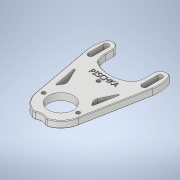
# Autodesk Inventor part: Motor Holder v3
Saved by Autodesk Inventor 2020.1 (Build 241239000, 239)
## iProperties
Created: 2019-03-01
Part Number: Motor Holder v3
Material: ABS Plastic
Document SubType Name: Modeling
Designer: Petar
Density: 1.06 g/cm^3
Appearance: Smooth - White
Mass: 12.2882 g
Surface Area: 69.5635 cm^2
Volume: 11.5927 cm^3
Author: Petar
Autodesk Inventor part; units mm, degrees
ref_plane "YZ Plane" through (0, 0, 0) normal (1, 0, 0) x (0, 1, 0)
ref_plane "XZ Plane" through (0, 0, 0) normal (0, 1, 0) x (-1, 0, 0)
ref_plane "XY Plane" through (0, 0, 0) normal (0, 0, 1) x (1, 0, 0)
sketch "Sketch1" plane through (0, 0, 0) normal (0, 1, 0) x (-1, 0, 0)
  line L0 (0, 0) -> (0, 51.5) construction
  circle A0 centre (0, 51.5) radius 10
  line L1 (16, -6.25) -> (16, 0)
  line L2 (21.5, 19.889372) -> (21.5, -14.110628) construction
  line L3 (-21.5, 18) -> (-21.5, -16) construction
  circle A1 centre (21.5, 3.5) radius 1.75 construction
  circle A2 centre (21.5, -3.5) radius 1.75 construction
  circle A3 centre (-21.5, 3.5) radius 1.75 construction
  circle A4 centre (-21.5, -3.5) radius 1.75 construction
  line L4 (-16, -6.25) -> (-16, 0)
  line L5 (21.5, 6.25) -> (21.5, -6.25) construction
  line L6 (19.45, 6.25) -> (19.45, -6.25)
  line L7 (23.55, -6.25) -> (23.55, 6.25)
  arc A5 (23.55, 6.25) -> (19.45, 6.25) centre (21.5, 6.25) ccw
  arc A6 (19.45, -6.25) -> (23.55, -6.25) centre (21.5, -6.25) ccw
  line L8 (-19.45, 6.25) -> (-19.45, -6.25)
  line L9 (-23.55, -6.25) -> (-23.55, 6.25)
  arc A7 (-19.45, 6.25) -> (-23.55, 6.25) centre (-21.5, 6.25) ccw
  arc A8 (-23.55, -6.25) -> (-19.45, -6.25) centre (-21.5, -6.25) ccw
  arc A9 (14.544724, 41.768556) -> (17.199681, 54.728155) centre (0, 51.5) ccw construction
  arc A10 (16, -6.25) -> (24.816002, -10.637953) centre (21.5, -6.25) ccw
  arc A11 (-24.816002, -10.637953) -> (-16, -6.25) centre (-21.5, -6.25) ccw
  line L10 (17.199681, 54.728155) -> (26.53665, 4.980583)
  line L11 (-17.199681, 54.728155) -> (-26.53665, 4.980583)
  circle A12 centre (0, 51.5) radius 13.75 construction
  circle A13 centre (9.722718, 61.222718) radius 1.5 construction
  circle A14 centre (9.722718, 41.777282) radius 1.5 construction
  line L12 (0, 51.5) -> (9.722718, 61.222718) construction
  line L13 (9.722718, 41.777282) -> (0, 51.5) construction
  circle A15 centre (-9.722718, 61.222718) radius 1.5 construction
  circle A16 centre (-9.722718, 41.777282) radius 1.5 construction
  circle A17 centre (13.75, 51.5) radius 1.5
  line L14 (13.75, 51.5) -> (0, 51.5) construction
  circle A18 centre (-13.75, 51.5) radius 1.5
  circle A19 centre (0, 21.442114) radius 1.5
  line L15 (14.544724, 41.768556) -> (18.735106, 19.442114)
  arc A20 (17.199681, 54.728155) -> (-17.199681, 54.728155) centre (0, 51.5) ccw
  arc A21 (-17.199681, 54.728155) -> (-14.544724, 41.768556) centre (0, 51.5) ccw construction
  line L16 (-14.544724, 41.768556) -> (-18.735106, 19.442114)
  line L17 (5, 68.27051) -> (0, 65.25) construction
  line L18 (0, 65.25) -> (-5, 68.27051) construction
  spline S0 degree 2 poles (5, 68.27051) (0, 65.25) (-5, 68.27051) knots 1 1 1 2 2 2
  line L19 (5, 68.27051) -> (-5, 68.27051) construction
  line L20 (18.735106, 19.442114) -> (-18.735106, 19.442114) construction
  line L21 (18.735106, 19.442114) -> (11.806239, 33.884362)
  line L22 (14.544724, 41.768556) -> (12.108743, 38.127711)
  arc A22 (12.108743, 38.127711) -> (11.806239, 33.884362) centre (15.676028, 35.740946) ccw
  line L23 (-18.735106, 19.442114) -> (-11.806239, 33.884362)
  line L24 (-14.544724, 41.768556) -> (-12.108743, 38.127711)
  arc A23 (-11.806239, 33.884362) -> (-12.108743, 38.127711) centre (-15.676028, 35.740946) ccw
  line L25 (14.298579, 19.442114) -> (8.163141, 32.230571) construction
  line L26 (14.298579, 19.442114) -> (7.49461, 25.938983) construction
  line L27 (8.163141, 32.230571) -> (6.995239, 30.485011) construction
  arc A24 (6.995239, 30.485011) -> (7.49461, 25.938983) centre (9.94862, 28.508992) ccw construction
  line L28 (-14.298579, 19.442114) -> (-8.163141, 32.230571) construction
  line L29 (-14.298579, 19.442114) -> (-7.49461, 25.938983) construction
  line L30 (-8.163141, 32.230571) -> (-6.995239, 30.485011) construction
  arc A25 (-7.49461, 25.938983) -> (-6.995239, 30.485011) centre (-9.94862, 28.508992) ccw construction
  arc A26 (24.816002, -10.637953) -> (27, 0) centre (0, 0) ccw
  arc A27 (-24.816002, -10.637953) -> (24.816002, -10.637953) centre (0, 0) ccw construction
  arc A28 (-10.270866, 24.970168) -> (-26.53665, 4.980583) centre (0, 0) ccw construction
  line L31 (21.5, -11.75) -> (-21.5, -11.75) construction
  line L32 (-21.213203, 69) -> (25, 69) construction
  line L33 (0, 65.25) -> (0, 61.5) construction
  arc A29 (13.760985, 8.163043) -> (-13.760985, 8.163043) centre (0, -11.5) ccw
  line L34 (13.760985, 8.163043) -> (-13.760985, 8.163043) construction
  arc A30 (16, 0) -> (13.760985, 8.163043) centre (0, 0) ccw
  arc A31 (-13.760985, 8.163043) -> (-16, 0) centre (0, 0) ccw
  arc A32 (27, 0) -> (26.53665, 4.980583) centre (0, 0) ccw
  arc A33 (-27, 0) -> (-24.816002, -10.637953) centre (0, 0) ccw
  arc A34 (-26.53665, 4.980583) -> (-27, 0) centre (0, 0) ccw
  arc A35 (26.53665, 4.980583) -> (-12.029232, 24.172248) centre (0, 0) ccw construction
  line L35 (16, 0) -> (-16, 0) construction
  point P0 (21.5, 0)
  point P1 (0, 12.5)
  dimension "d1" = 20
  dimension "d0" = 51.5
  dimension "d3" = 3.5
  dimension "d4" = 3.5
  dimension "d5" = 7
  dimension "d9" = 3.5
  dimension "d11" = 32
  dimension "d15" = 4.1
  dimension "d24" = 3
  dimension "d25" = 3
  dimension "d27" = 45
  dimension "d29" = 3
  dimension "d30" = 3
  dimension "d50" = 10
  dimension "d53" = 27
  dimension "d75" = 80.75
  dimension "d76" = 7.5
  dimension "d77" = 3.75
  dimension "d81" = 6.25
  dimension "d82" = 12.5
  dimension "d85" = 5
  dimension "d86" = 4
  dimension "d98" = 15
  dimension "d99" = 24
  dimension "d102" = 43
  dimension "d103" = 2
  constraints: 70 end point, 59 point on circle, 35 centre point, 26 symmetric about line, 19 tangent, 13 point on line, 7 coincident, 5 horizontal, 5 vertical, 3 parallel, 2 perpendicular, 1 collinear, 1 midpoint, 1 vertical alignment, 16 other
  measures "d0" distance of L0.start L0.end
  measures "d3" diameter of A1
  measures "d4" diameter of A2
  measures "d5" distance of A2.centre A1.centre
  measures "d9" vertical distance of L0.start A1.centre
  measures "d11" distance between parallel lines of L4 L1
  measures "d15" distance between parallel lines of L6 L7
  measures "d24" diameter of A13
  measures "d25" diameter of A14
  measures "d27" angle of L0 L13
  measures "d29" diameter of A17
  measures "d30" diameter of A19
  measures "d50" distance of L17.start L18.end
  measures "d53" radius of A26
  measures "d75" distance between parallel lines of L31 L32
  measures "d81" vertical distance of L5.start point (0, 12.5)
  measures "d82" distance of L5.end L5.start
  measures "d85" distance between parallel lines of L10 L15
  measures "d86" distance between parallel lines of L21 L25
  measures "d98" angle of L15 L21
  measures "d99" radius of A29
  measures "d102" distance of A4.centre A2.centre
  measures "d103" distance from line of A19.centre L20
extrude "Extrusion3" add sketch "Sketch1" along normal blind 5.5 contours L1 A30 A29 A31 L4 A11 A33 A34 L11 A20 S0 L10 A32 A26 A10
thread "Thread1" size "M3x0.5" class "6H" standard "ANSI Metric M Profile" full length
thread "Thread2" size "M3x0.5" class "6H" standard "ANSI Metric M Profile" full length
thread "Thread3" size "M3x0.5" class "6H" standard "ANSI Metric M Profile" full length
sketch "Sketch3" plane through (0, 5.5, 0) normal (0, 1, 0) x (1, 0, 0)
  line L0 (-12.5, -14.442114) -> (12.5, -14.442114) construction
  line L1 (12.5, -14.442114) -> (12.5, -19.442114) construction
  line L2 (12.5, -19.442114) -> (-12.5, -19.442114) construction
  line L3 (-12.5, -19.442114) -> (-12.5, -14.442114) construction
  line L4 (0, 0) -> (0, -51.5) construction
  circle A0 centre (0, -21.442114) radius 1.5
  circle A1 centre (0, -51.5) radius 10 construction
  arc A2 (-24.816002, 10.637953) -> (-26.53665, -4.980583) centre (0, 0) ccw construction
  spline S0 degree 2 poles (-7.943274, -16.147949) (-7.943274, -16.407268) (-8.128039, -16.874043) (-8.293355, -17.036118) knots 0 0 0 1 2 2 2
  spline S1 degree 2 poles (-8.293355, -17.036118) (-8.500811, -17.240332) (-9.061589, -17.451029) (-9.489465, -17.451029) knots 0 0 0 1 2 2 2
  line L5 (-9.489465, -17.451029) -> (-9.940033, -17.451029)
  line L6 (-9.940033, -17.451029) -> (-9.940033, -18.942114)
  line L7 (-9.940033, -18.942114) -> (-10.471637, -18.942114)
  line L8 (-10.471637, -18.942114) -> (-10.471637, -14.942114)
  line L9 (-10.471637, -14.942114) -> (-9.466775, -14.942114)
  spline S2 degree 2 poles (-9.466775, -14.942114) (-9.110211, -14.942114) (-8.611021, -15.058808) (-8.419773, -15.191709) knots 0 0 0 1 2 2 2
  spline S3 degree 2 poles (-8.419773, -15.191709) (-8.19611, -15.344059) (-7.943274, -15.814076) (-7.943274, -16.147949) knots 0 0 0 1 2 2 2
  spline S4 degree 2 poles (-8.497569, -16.164157) (-8.497569, -15.956701) (-8.640195, -15.652001) (-8.786062, -15.554756) knots 0 0 0 1 2 2 2
  spline S5 degree 2 poles (-8.786062, -15.554756) (-8.91248, -15.470477) (-9.249595, -15.402406) (-9.49919, -15.402406) knots 0 0 0 1 2 2 2
  line L10 (-9.49919, -15.402406) -> (-9.940033, -15.402406)
  line L11 (-9.940033, -15.402406) -> (-9.940033, -16.99722)
  line L12 (-9.940033, -16.99722) -> (-9.576986, -16.99722)
  spline S6 degree 2 poles (-9.576986, -16.99722) (-9.252837, -16.99722) (-8.854133, -16.893492) (-8.724474, -16.757349) knots 0 0 0 1 2 2 2
  spline S7 degree 2 poles (-8.724474, -16.757349) (-8.604538, -16.637414) (-8.497569, -16.355405) (-8.497569, -16.164157) knots 0 0 0 1 2 2 2
  line L13 (-6.04376, -18.942114) -> (-7.593193, -18.942114)
  line L14 (-7.593193, -18.942114) -> (-7.593193, -18.533687)
  line L15 (-7.593193, -18.533687) -> (-7.084279, -18.533687)
  line L16 (-7.084279, -18.533687) -> (-7.084279, -15.350542)
  line L17 (-7.084279, -15.350542) -> (-7.593193, -15.350542)
  line L18 (-7.593193, -15.350542) -> (-7.593193, -14.942114)
  line L19 (-7.593193, -14.942114) -> (-6.04376, -14.942114)
  line L20 (-6.04376, -14.942114) -> (-6.04376, -15.350542)
  line L21 (-6.04376, -15.350542) -> (-6.552674, -15.350542)
  line L22 (-6.552674, -15.350542) -> (-6.552674, -18.533687)
  line L23 (-6.552674, -18.533687) -> (-6.04376, -18.533687)
  line L24 (-6.04376, -18.533687) -> (-6.04376, -18.942114)
  spline S8 degree 2 poles (-4.270665, -19.013427) (-4.705025, -19.013427) (-5.314425, -18.831904) (-5.583469, -18.702244) knots 0 0 0 1 2 2 2
  line L25 (-5.583469, -18.702244) -> (-5.583469, -18.034497)
  line L26 (-5.583469, -18.034497) -> (-5.544571, -18.034497)
  spline S9 degree 2 poles (-5.544571, -18.034497) (-5.28201, -18.28085) (-4.617504, -18.553136) (-4.309563, -18.553136) knots 0 0 0 1 2 2 2
  spline S10 degree 2 poles (-4.309563, -18.553136) (-3.86872, -18.553136) (-3.418153, -18.186847) (-3.418153, -17.885388) knots 0 0 0 1 2 2 2
  spline S11 degree 2 poles (-3.418153, -17.885388) (-3.418153, -17.645518) (-3.654781, -17.347301) (-3.910859, -17.272747) knots 0 0 0 1 2 2 2
  spline S12 degree 2 poles (-3.910859, -17.272747) (-4.095624, -17.220883) (-4.403566, -17.14957) (-4.633712, -17.091223) knots 0 0 0 1 2 2 2
  spline S13 degree 2 poles (-4.633712, -17.091223) (-4.841167, -17.036118) (-5.168558, -16.870802) (-5.294976, -16.7379) knots 0 0 0 1 2 2 2
  spline S14 degree 2 poles (-5.294976, -16.7379) (-5.418153, -16.604999) (-5.554295, -16.248435) (-5.554295, -16.015048) knots 0 0 0 1 2 2 2
  spline S15 degree 2 poles (-5.554295, -16.015048) (-5.554295, -15.528824) (-4.795786, -14.870802) (-4.209076, -14.870802) knots 0 0 0 1 2 2 2
  spline S16 degree 2 poles (-4.209076, -14.870802) (-3.871961, -14.870802) (-3.275527, -15.003703) (-3.019449, -15.130121) knots 0 0 0 1 2 2 2
  line L27 (-3.019449, -15.130121) -> (-3.019449, -15.765453)
  line L28 (-3.019449, -15.765453) -> (-3.058347, -15.765453)
  spline S17 degree 2 poles (-3.058347, -15.765453) (-3.249595, -15.590413) (-3.846029, -15.331093) (-4.17342, -15.331093) knots 0 0 0 1 2 2 2
  spline S18 degree 2 poles (-4.17342, -15.331093) (-4.54295, -15.331093) (-5, -15.677933) (-5, -15.959943) knots 0 0 0 1 2 2 2
  spline S19 degree 2 poles (-5, -15.959943) (-5, -16.212779) (-4.730956, -16.514238) (-4.47812, -16.582309) knots 0 0 0 1 2 2 2
  spline S20 degree 2 poles (-4.47812, -16.582309) (-4.309563, -16.62769) (-3.820097, -16.744383) (-3.658023, -16.793006) knots 0 0 0 1 2 2 2
  spline S21 degree 2 poles (-3.658023, -16.793006) (-3.246354, -16.919424) (-2.863858, -17.428338) (-2.863858, -17.80111) knots 0 0 0 1 2 2 2
  spline S22 degree 2 poles (-2.863858, -17.80111) (-2.863858, -18.037738) (-3.055106, -18.491547) (-3.226905, -18.65038) knots 0 0 0 1 2 2 2
  spline S23 degree 2 poles (-3.226905, -18.65038) (-3.418153, -18.825421) (-3.904376, -19.013427) (-4.270665, -19.013427) knots 0 0 0 1 2 2 2
  spline S24 degree 2 poles (-0.76013, -19.013427) (-1.149109, -19.013427) (-1.807131, -18.750866) (-2.047002, -18.488306) knots 0 0 0 1 2 2 2
  spline S25 degree 2 poles (-2.047002, -18.488306) (-2.286872, -18.228986) (-2.549433, -17.451029) (-2.549433, -16.945356) knots 0 0 0 1 2 2 2
  spline S26 degree 2 poles (-2.549433, -16.945356) (-2.549433, -16.442925) (-2.293355, -15.697382) (-2.050243, -15.421855) knots 0 0 0 1 2 2 2
  spline S27 degree 2 poles (-2.050243, -15.421855) (-1.810373, -15.152811) (-1.155592, -14.870802) (-0.750405, -14.870802) knots 0 0 0 1 2 2 2
  spline S28 degree 2 poles (-0.750405, -14.870802) (-0.549433, -14.870802) (-0.19611, -14.929148) (-0.047002, -14.974529) knots 0 0 0 1 2 2 2
  spline S29 degree 2 poles (-0.047002, -14.974529) (0.082658, -15.016669) (0.351702, -15.136604) (0.484603, -15.207917) knots 0 0 0 1 2 2 2
  line L29 (0.484603, -15.207917) -> (0.484603, -15.849732)
  line L30 (0.484603, -15.849732) -> (0.442463, -15.849732)
  spline S30 degree 2 poles (0.442463, -15.849732) (0.371151, -15.784902) (0.150729, -15.603379) (-0.008104, -15.515858) knots 0 0 0 1 2 2 2
  spline S31 degree 2 poles (-0.008104, -15.515858) (-0.160454, -15.43158) (-0.520259, -15.32461) (-0.753647, -15.32461) knots 0 0 0 1 2 2 2
  spline S32 degree 2 poles (-0.753647, -15.32461) (-1.009725, -15.32461) (-1.466775, -15.535307) (-1.638574, -15.73628) knots 0 0 0 1 2 2 2
  spline S33 degree 2 poles (-1.638574, -15.73628) (-1.807131, -15.940494) (-1.995138, -16.559618) (-1.995138, -16.945356) knots 0 0 0 1 2 2 2
  spline S34 degree 2 poles (-1.995138, -16.945356) (-1.995138, -17.357025) (-1.797407, -17.950218) (-1.625608, -18.154432) knots 0 0 0 1 2 2 2
  spline S35 degree 2 poles (-1.625608, -18.154432) (-1.45705, -18.352163) (-1.006483, -18.553136) (-0.753647, -18.553136) knots 0 0 0 1 2 2 2
  spline S36 degree 2 poles (-0.753647, -18.553136) (-0.523501, -18.553136) (-0.131281, -18.439683) (0.02107, -18.355405) knots 0 0 0 1 2 2 2
  spline S37 degree 2 poles (0.02107, -18.355405) (0.166937, -18.271126) (0.384117, -18.096085) (0.445705, -18.034497) knots 0 0 0 1 2 2 2
  line L31 (0.445705, -18.034497) -> (0.484603, -18.034497)
  line L32 (0.484603, -18.034497) -> (0.484603, -18.669829)
  spline S38 degree 2 poles (0.484603, -18.669829) (0.351702, -18.731418) (0.118314, -18.84487) (-0.047002, -18.896734) knots 0 0 0 1 2 2 2
  spline S39 degree 2 poles (-0.047002, -18.896734) (-0.222042, -18.95508) (-0.520259, -19.013427) (-0.76013, -19.013427) knots 0 0 0 1 2 2 2
  line L33 (3.884927, -18.942114) -> (3.353322, -18.942114)
  line L34 (3.353322, -18.942114) -> (3.353322, -16.984254)
  line L35 (3.353322, -16.984254) -> (1.512155, -16.984254)
  line L36 (1.512155, -16.984254) -> (1.512155, -18.942114)
  line L37 (1.512155, -18.942114) -> (0.980551, -18.942114)
  line L38 (0.980551, -18.942114) -> (0.980551, -14.942114)
  line L39 (0.980551, -14.942114) -> (1.512155, -14.942114)
  line L40 (1.512155, -14.942114) -> (1.512155, -16.510996)
  line L41 (1.512155, -16.510996) -> (3.353322, -16.510996)
  line L42 (3.353322, -16.510996) -> (3.353322, -14.942114)
  line L43 (3.353322, -14.942114) -> (3.884927, -14.942114)
  line L44 (3.884927, -14.942114) -> (3.884927, -18.942114)
  line L45 (7.612642, -18.942114) -> (6.922204, -18.942114)
  line L46 (6.922204, -18.942114) -> (5.460292, -17.081499)
  line L47 (5.460292, -17.081499) -> (5.226904, -17.344059)
  line L48 (5.226904, -17.344059) -> (5.226904, -18.942114)
  line L49 (5.226904, -18.942114) -> (4.6953, -18.942114)
  line L50 (4.6953, -18.942114) -> (4.6953, -14.942114)
  line L51 (4.6953, -14.942114) -> (5.226904, -14.942114)
  line L52 (5.226904, -14.942114) -> (5.226904, -16.78004)
  line L53 (5.226904, -16.78004) -> (6.867099, -14.942114)
  line L54 (6.867099, -14.942114) -> (7.515397, -14.942114)
  line L55 (7.515397, -14.942114) -> (5.858995, -16.728176)
  line L56 (5.858995, -16.728176) -> (7.612642, -18.942114)
  line L57 (7.49919, -18.942114) -> (8.84765, -14.942114)
  line L58 (8.84765, -14.942114) -> (9.502431, -14.942114)
  line L59 (9.502431, -14.942114) -> (10.850891, -18.942114)
  line L60 (10.850891, -18.942114) -> (10.290113, -18.942114)
  line L61 (10.290113, -18.942114) -> (9.927066, -17.8238)
  line L62 (9.927066, -17.8238) -> (8.400324, -17.8238)
  line L63 (8.400324, -17.8238) -> (8.037277, -18.942114)
  line L64 (8.037277, -18.942114) -> (7.49919, -18.942114)
  line L65 (9.781199, -17.369991) -> (9.162075, -15.486685)
  line L66 (9.162075, -15.486685) -> (8.546191, -17.369991)
  line L67 (8.546191, -17.369991) -> (9.781199, -17.369991)
  dimension "d68" = 2
  dimension "d69" = 5
  dimension "d70" = 25
  constraints: 3 end point, 1 coincident, 1 vertical, 3 other
  measures "d68" distance from line of L2 A0.centre
  measures "d69" distance between parallel lines of L0 L2
  measures "d70" distance between parallel lines of L3 L1
emboss "Emboss1" sketch "Sketch3" operation cut depth 0.2 direction (0, -1, 0) contours S0 S1 L5 L6 L7 L8 L9 S2 S3 | L13 L14 L15 L16 L17 L18 L19 L20 L21 L22 L23 L24 | S8 L25 L26 S9 S10 S11 S12 S13 S14 S15 S16 L27 L28 S17 S18 S19 S20 S21 S22 S23 | S24 S25 S26 S27 S28 S29 L29 L30 S30 S31 S32 S33 S34 S35 S36 S37 L31 L32 S38 S39 | L33 L34 L35 L36 L37 L38 L39 L40 L41 L42 L43 L44 | L45 L57 L56 | L56 L57 L58 L59 L60 L61 L62 L63 L64 | L45 L46 L47 L48 L49 L50 L51 L52 L53 L54 L55 L56 L57
sketch "Sketch4" plane through (0, 0, 0) normal (0, -1, 0) x (1, 0, 0)
  circle A0 centre (0, 21.442114) radius 1.5
  line L0 (12.5, 14.442114) -> (-12.5, 14.442114) construction
  line L1 (-12.5, 14.442114) -> (-12.5, 19.442114) construction
  line L2 (-12.5, 19.442114) -> (12.5, 19.442114) construction
  line L3 (12.5, 19.442114) -> (12.5, 14.442114) construction
  arc A1 (24.816002, -10.637953) -> (26.53665, 4.980583) centre (0, 0) ccw construction
  circle A2 centre (0, 51.5) radius 10 construction
  line L4 (0, 0) -> (0, 51.5) construction
  spline S0 degree 2 poles (7.943274, 16.147949) (7.943274, 16.407268) (8.128039, 16.874043) (8.293355, 17.036118) knots 0 0 0 1 2 2 2
  spline S1 degree 2 poles (8.293355, 17.036118) (8.500811, 17.240332) (9.061589, 17.451029) (9.489465, 17.451029) knots 0 0 0 1 2 2 2
  line L5 (9.489465, 17.451029) -> (9.940033, 17.451029)
  line L6 (9.940033, 17.451029) -> (9.940033, 18.942114)
  line L7 (9.940033, 18.942114) -> (10.471637, 18.942114)
  line L8 (10.471637, 18.942114) -> (10.471637, 14.942114)
  line L9 (10.471637, 14.942114) -> (9.466775, 14.942114)
  spline S2 degree 2 poles (9.466775, 14.942114) (9.110211, 14.942114) (8.611021, 15.058808) (8.419773, 15.191709) knots 0 0 0 1 2 2 2
  spline S3 degree 2 poles (8.419773, 15.191709) (8.19611, 15.344059) (7.943274, 15.814076) (7.943274, 16.147949) knots 0 0 0 1 2 2 2
  spline S4 degree 2 poles (8.497569, 16.164157) (8.497569, 15.956701) (8.640195, 15.652001) (8.786062, 15.554756) knots 0 0 0 1 2 2 2
  spline S5 degree 2 poles (8.786062, 15.554756) (8.91248, 15.470477) (9.249595, 15.402406) (9.49919, 15.402406) knots 0 0 0 1 2 2 2
  line L10 (9.49919, 15.402406) -> (9.940033, 15.402406)
  line L11 (9.940033, 15.402406) -> (9.940033, 16.99722)
  line L12 (9.940033, 16.99722) -> (9.576986, 16.99722)
  spline S6 degree 2 poles (9.576986, 16.99722) (9.252837, 16.99722) (8.854133, 16.893492) (8.724474, 16.757349) knots 0 0 0 1 2 2 2
  spline S7 degree 2 poles (8.724474, 16.757349) (8.604538, 16.637414) (8.497569, 16.355405) (8.497569, 16.164157) knots 0 0 0 1 2 2 2
  line L13 (6.04376, 18.942114) -> (7.593193, 18.942114)
  line L14 (7.593193, 18.942114) -> (7.593193, 18.533687)
  line L15 (7.593193, 18.533687) -> (7.084279, 18.533687)
  line L16 (7.084279, 18.533687) -> (7.084279, 15.350542)
  line L17 (7.084279, 15.350542) -> (7.593193, 15.350542)
  line L18 (7.593193, 15.350542) -> (7.593193, 14.942114)
  line L19 (7.593193, 14.942114) -> (6.04376, 14.942114)
  line L20 (6.04376, 14.942114) -> (6.04376, 15.350542)
  line L21 (6.04376, 15.350542) -> (6.552674, 15.350542)
  line L22 (6.552674, 15.350542) -> (6.552674, 18.533687)
  line L23 (6.552674, 18.533687) -> (6.04376, 18.533687)
  line L24 (6.04376, 18.533687) -> (6.04376, 18.942114)
  spline S8 degree 2 poles (4.270665, 19.013427) (4.705025, 19.013427) (5.314425, 18.831904) (5.583469, 18.702244) knots 0 0 0 1 2 2 2
  line L25 (5.583469, 18.702244) -> (5.583469, 18.034497)
  line L26 (5.583469, 18.034497) -> (5.544571, 18.034497)
  spline S9 degree 2 poles (5.544571, 18.034497) (5.28201, 18.28085) (4.617504, 18.553136) (4.309563, 18.553136) knots 0 0 0 1 2 2 2
  spline S10 degree 2 poles (4.309563, 18.553136) (3.86872, 18.553136) (3.418153, 18.186847) (3.418153, 17.885388) knots 0 0 0 1 2 2 2
  spline S11 degree 2 poles (3.418153, 17.885388) (3.418153, 17.645518) (3.654781, 17.347301) (3.910859, 17.272747) knots 0 0 0 1 2 2 2
  spline S12 degree 2 poles (3.910859, 17.272747) (4.095624, 17.220883) (4.403566, 17.14957) (4.633712, 17.091223) knots 0 0 0 1 2 2 2
  spline S13 degree 2 poles (4.633712, 17.091223) (4.841167, 17.036118) (5.168558, 16.870802) (5.294976, 16.7379) knots 0 0 0 1 2 2 2
  spline S14 degree 2 poles (5.294976, 16.7379) (5.418153, 16.604999) (5.554295, 16.248435) (5.554295, 16.015048) knots 0 0 0 1 2 2 2
  spline S15 degree 2 poles (5.554295, 16.015048) (5.554295, 15.528824) (4.795786, 14.870802) (4.209076, 14.870802) knots 0 0 0 1 2 2 2
  spline S16 degree 2 poles (4.209076, 14.870802) (3.871961, 14.870802) (3.275527, 15.003703) (3.019449, 15.130121) knots 0 0 0 1 2 2 2
  line L27 (3.019449, 15.130121) -> (3.019449, 15.765453)
  line L28 (3.019449, 15.765453) -> (3.058347, 15.765453)
  spline S17 degree 2 poles (3.058347, 15.765453) (3.249595, 15.590413) (3.846029, 15.331093) (4.17342, 15.331093) knots 0 0 0 1 2 2 2
  spline S18 degree 2 poles (4.17342, 15.331093) (4.54295, 15.331093) (5, 15.677933) (5, 15.959943) knots 0 0 0 1 2 2 2
  spline S19 degree 2 poles (5, 15.959943) (5, 16.212779) (4.730956, 16.514238) (4.47812, 16.582309) knots 0 0 0 1 2 2 2
  spline S20 degree 2 poles (4.47812, 16.582309) (4.309563, 16.62769) (3.820097, 16.744383) (3.658023, 16.793006) knots 0 0 0 1 2 2 2
  spline S21 degree 2 poles (3.658023, 16.793006) (3.246354, 16.919424) (2.863858, 17.428338) (2.863858, 17.80111) knots 0 0 0 1 2 2 2
  spline S22 degree 2 poles (2.863858, 17.80111) (2.863858, 18.037738) (3.055106, 18.491547) (3.226905, 18.65038) knots 0 0 0 1 2 2 2
  spline S23 degree 2 poles (3.226905, 18.65038) (3.418153, 18.825421) (3.904376, 19.013427) (4.270665, 19.013427) knots 0 0 0 1 2 2 2
  spline S24 degree 2 poles (0.76013, 19.013427) (1.149109, 19.013427) (1.807131, 18.750866) (2.047002, 18.488306) knots 0 0 0 1 2 2 2
  spline S25 degree 2 poles (2.047002, 18.488306) (2.286872, 18.228986) (2.549433, 17.451029) (2.549433, 16.945356) knots 0 0 0 1 2 2 2
  spline S26 degree 2 poles (2.549433, 16.945356) (2.549433, 16.442925) (2.293355, 15.697382) (2.050243, 15.421855) knots 0 0 0 1 2 2 2
  spline S27 degree 2 poles (2.050243, 15.421855) (1.810373, 15.152811) (1.155592, 14.870802) (0.750405, 14.870802) knots 0 0 0 1 2 2 2
  spline S28 degree 2 poles (0.750405, 14.870802) (0.549433, 14.870802) (0.19611, 14.929148) (0.047002, 14.974529) knots 0 0 0 1 2 2 2
  spline S29 degree 2 poles (0.047002, 14.974529) (-0.082658, 15.016669) (-0.351702, 15.136604) (-0.484603, 15.207917) knots 0 0 0 1 2 2 2
  line L29 (-0.484603, 15.207917) -> (-0.484603, 15.849732)
  line L30 (-0.484603, 15.849732) -> (-0.442463, 15.849732)
  spline S30 degree 2 poles (-0.442463, 15.849732) (-0.371151, 15.784902) (-0.150729, 15.603379) (0.008104, 15.515858) knots 0 0 0 1 2 2 2
  spline S31 degree 2 poles (0.008104, 15.515858) (0.160454, 15.43158) (0.520259, 15.32461) (0.753647, 15.32461) knots 0 0 0 1 2 2 2
  spline S32 degree 2 poles (0.753647, 15.32461) (1.009725, 15.32461) (1.466775, 15.535307) (1.638574, 15.73628) knots 0 0 0 1 2 2 2
  spline S33 degree 2 poles (1.638574, 15.73628) (1.807131, 15.940494) (1.995138, 16.559618) (1.995138, 16.945356) knots 0 0 0 1 2 2 2
  spline S34 degree 2 poles (1.995138, 16.945356) (1.995138, 17.357025) (1.797407, 17.950218) (1.625608, 18.154432) knots 0 0 0 1 2 2 2
  spline S35 degree 2 poles (1.625608, 18.154432) (1.45705, 18.352163) (1.006483, 18.553136) (0.753647, 18.553136) knots 0 0 0 1 2 2 2
  spline S36 degree 2 poles (0.753647, 18.553136) (0.523501, 18.553136) (0.131281, 18.439683) (-0.02107, 18.355405) knots 0 0 0 1 2 2 2
  spline S37 degree 2 poles (-0.02107, 18.355405) (-0.166937, 18.271126) (-0.384117, 18.096085) (-0.445705, 18.034497) knots 0 0 0 1 2 2 2
  line L31 (-0.445705, 18.034497) -> (-0.484603, 18.034497)
  line L32 (-0.484603, 18.034497) -> (-0.484603, 18.669829)
  spline S38 degree 2 poles (-0.484603, 18.669829) (-0.351702, 18.731418) (-0.118314, 18.84487) (0.047002, 18.896734) knots 0 0 0 1 2 2 2
  spline S39 degree 2 poles (0.047002, 18.896734) (0.222042, 18.95508) (0.520259, 19.013427) (0.76013, 19.013427) knots 0 0 0 1 2 2 2
  line L33 (-3.884927, 18.942114) -> (-3.353322, 18.942114)
  line L34 (-3.353322, 18.942114) -> (-3.353322, 16.984254)
  line L35 (-3.353322, 16.984254) -> (-1.512155, 16.984254)
  line L36 (-1.512155, 16.984254) -> (-1.512155, 18.942114)
  line L37 (-1.512155, 18.942114) -> (-0.980551, 18.942114)
  line L38 (-0.980551, 18.942114) -> (-0.980551, 14.942114)
  line L39 (-0.980551, 14.942114) -> (-1.512155, 14.942114)
  line L40 (-1.512155, 14.942114) -> (-1.512155, 16.510996)
  line L41 (-1.512155, 16.510996) -> (-3.353322, 16.510996)
  line L42 (-3.353322, 16.510996) -> (-3.353322, 14.942114)
  line L43 (-3.353322, 14.942114) -> (-3.884927, 14.942114)
  line L44 (-3.884927, 14.942114) -> (-3.884927, 18.942114)
  line L45 (-7.612642, 18.942114) -> (-6.922204, 18.942114)
  line L46 (-6.922204, 18.942114) -> (-5.460292, 17.081499)
  line L47 (-5.460292, 17.081499) -> (-5.226904, 17.344059)
  line L48 (-5.226904, 17.344059) -> (-5.226904, 18.942114)
  line L49 (-5.226904, 18.942114) -> (-4.6953, 18.942114)
  line L50 (-4.6953, 18.942114) -> (-4.6953, 14.942114)
  line L51 (-4.6953, 14.942114) -> (-5.226904, 14.942114)
  line L52 (-5.226904, 14.942114) -> (-5.226904, 16.78004)
  line L53 (-5.226904, 16.78004) -> (-6.867099, 14.942114)
  line L54 (-6.867099, 14.942114) -> (-7.515397, 14.942114)
  line L55 (-7.515397, 14.942114) -> (-5.858995, 16.728176)
  line L56 (-5.858995, 16.728176) -> (-7.612642, 18.942114)
  line L57 (-7.49919, 18.942114) -> (-8.84765, 14.942114)
  line L58 (-8.84765, 14.942114) -> (-9.502431, 14.942114)
  line L59 (-9.502431, 14.942114) -> (-10.850891, 18.942114)
  line L60 (-10.850891, 18.942114) -> (-10.290113, 18.942114)
  line L61 (-10.290113, 18.942114) -> (-9.927066, 17.8238)
  line L62 (-9.927066, 17.8238) -> (-8.400324, 17.8238)
  line L63 (-8.400324, 17.8238) -> (-8.037277, 18.942114)
  line L64 (-8.037277, 18.942114) -> (-7.49919, 18.942114)
  line L65 (-9.781199, 17.369991) -> (-9.162075, 15.486685)
  line L66 (-9.162075, 15.486685) -> (-8.546191, 17.369991)
  line L67 (-8.546191, 17.369991) -> (-9.781199, 17.369991)
  dimension "d67" = 2
  dimension "d71" = 5
  dimension "d72" = 25
  constraints: 2 end point, 1 vertical, 3 other
  measures "d67" distance from line of L2 A0.centre
  measures "d71" distance between parallel lines of L2 L0
  measures "d72" distance between parallel lines of L3 L1
emboss "Emboss2" sketch "Sketch4" operation cut depth 0.2 direction (0, 1, 0) contours S0 S1 L5 L6 L7 L8 L9 S2 S3 | L13 L14 L15 L16 L17 L18 L19 L20 L21 L22 L23 L24 | S8 L25 L26 S9 S10 S11 S12 S13 S14 S15 S16 L27 L28 S17 S18 S19 S20 S21 S22 S23 | S24 S25 S26 S27 S28 S29 L29 L30 S30 S31 S32 S33 S34 S35 S36 S37 L31 L32 S38 S39 | L33 L34 L35 L36 L37 L38 L39 L40 L41 L42 L43 L44 | L45 L57 L56 | L56 L57 L58 L59 L60 L61 L62 L63 L64 | L45 L46 L47 L48 L49 L50 L51 L52 L53 L54 L55 L56 L57
fillet "Fillet3" radius 0.5 4 edges at (-18.7351, 2.75, 19.4421) (-14.5447, 2.75, 41.7686) (14.5447, 2.75, 41.7686) (18.7351, 2.75, 19.4421)
fillet "Fillet5" radius 2 6 edges at (-5, 2.75, 68.2705) (5, 2.75, 68.2705) (24.816, 2.75, -10.638) (-24.816, 2.75, -10.638) (-13.761, 2.75, 8.163) (13.761, 2.75, 8.163)
chamfer "Chamfer3" distance 0.5 angle 45 40 edges at (13.3091, 5.5, 62.863) (21.8682, 5.5, 29.8544) (26.8705, 5.5, -2.6415) (24.7034, 5.5, -10.6299) (18.713, 5.5, -10.9916) (16, 5.5, -3.125) (15.4929, 5.5, 3.9962) (13.7269, 5.5, 8.124) (0, 5.5, 12.5) (5.0769, 5.5, 68.0928) (0, 5.5, 66.7603) (-5.0769, 5.5, 68.0928) (-13.3091, 5.5, 62.863) (-21.8682, 5.5, 29.8544) (-26.8705, 5.5, -2.6415) (-24.7034, 5.5, -10.6299) (-18.713, 5.5, -10.9916) (-16, 5.5, -3.125) (-15.4929, 5.5, 3.9962) (-13.7269, 5.5, 8.124) (0, 0, 66.7603) (5.0769, 0, 68.0928) (13.3091, 0, 62.863) (21.8682, 0, 29.8544) (26.8705, 0, -2.6415) (24.7034, 0, -10.6299) (18.713, 0, -10.9916) (16, 0, -3.125) (15.4929, 0, 3.9962) (13.7269, 0, 8.124) (0, 0, 12.5) (-5.0769, 0, 68.0928) (-13.3091, 0, 62.863) (-21.8682, 0, 29.8544) (-26.8705, 0, -2.6415) (-24.7034, 0, -10.6299) (-18.713, 0, -10.9916) (-16, 0, -3.125) (-15.4929, 0, 3.9962) (-13.7269, 0, 8.124)
sketch "Center Lines" plane through (0, 5.5, 0) normal (0, 1, 0) x (1, 0, 0)
  circle A0 centre (21.242, -3.5) radius 1.666
  circle A1 centre (21.242, 3.5) radius 1.666
  circle A2 centre (-21.242, -3.5) radius 1.666
  circle A3 centre (-21.242, 3.5) radius 1.666
  line L0 (21.242, -3.5) -> (21.242, 3.5) construction
  line L1 (-21.242, -3.5) -> (-21.242, 3.5) construction
  line L2 (21.5, -3.5) -> (-21.5, -3.5) construction
  circle A4 centre (0, -51.5) radius 10 construction
  line L3 (0, -51.5) -> (0, 0) construction
  dimension "d109" = 7
  dimension "d110" = 7
  dimension "d113" = 3.332
  dimension "d115" = 42.484
  constraints: 8 end point, 4 centre point, 3 equal radius, 3 vertical, 2 point on line, 1 horizontal, 1 perpendicular, 1 other
  measures "d109" distance of L1.start L1.end
  measures "d110" distance of L0.start L0.end
  measures "d113" diameter of A0
  measures "d115" distance between parallel lines of L1 L0
body "Solid3"
